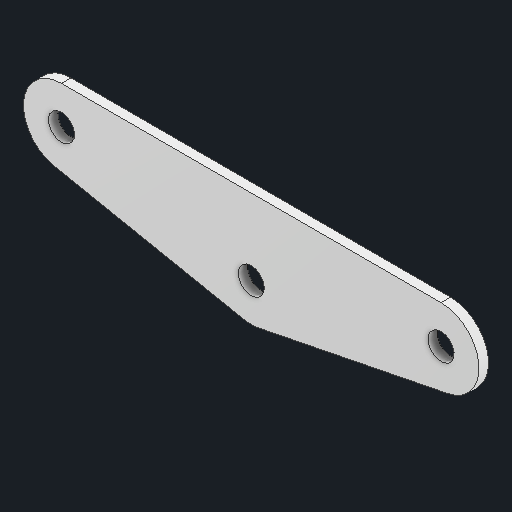
# Autodesk Inventor part: gearbox_gusset
Saved by Autodesk Inventor 2025 (Build 290162000, 162)
## iProperties
Created: 2024-06-27
Part Number: gearbox_gusset
Material: Acetal Resin, White
Document SubType Name: Modeling
Designer: Averey Ku
Density: 1.425 g/cm^3
Appearance: Smooth - White
Author: Averey Ku
Autodesk Inventor part; units mm, degrees
ref_plane "YZ Plane" through (0, 0, 0) normal (1, 0, 0) x (0, 1, 0)
ref_plane "XZ Plane" through (0, 0, 0) normal (0, 1, 0) x (-1, 0, 0)
ref_plane "XY Plane" through (0, 0, 0) normal (0, 0, 1) x (1, 0, 0)
sketch "main" plane through (0, 0, 0) normal (0, 0, 1) x (1, 0, 0)
  circle A0 centre (5.5393, 31.9986) radius 2.1844
  circle A1 centre (5.5393, -31.5014) radius 2.1844
  arc A2 (11.8893, 31.9986) -> (-0.6874, 33.244) centre (5.5393, 31.9986) ccw
  arc A3 (-0.6874, -32.7467) -> (11.8893, -31.5014) centre (5.5393, -31.5014) ccw
  line L0 (11.8893, 31.9986) -> (11.8893, -31.5014)
  circle A4 centre (-0.8107, 0.2486) radius 2.1844
  arc A5 (-7.0374, 1.494) -> (-7.0374, -0.9967) centre (-0.8107, 0.2486) ccw
  line L1 (-0.6874, 33.244) -> (-7.0374, 1.494)
  line L2 (-7.0374, -0.9967) -> (-0.6874, -32.7467)
  point P0 (2.0663, 0.2486)
sketch "Sketch1" plane through (0, 0, 0) normal (0, 0, 1) x (1, 0, 0)
  circle A0 centre (0, 0) radius 2.1844
  circle A1 centre (63.5, -0.0173) radius 2.1844
  arc A2 (0.0017, 6.35) -> (-1.247, -6.2263) centre (0, 0) ccw
  arc A3 (64.7436, -6.2443) -> (63.5017, 6.3327) centre (63.5, -0.0173) ccw
  line L0 (0.0017, 6.35) -> (63.5017, 6.3327)
  circle A4 centre (31.7483, -6.3586) radius 2.1844
  arc A5 (30.5012, -12.585) -> (32.9919, -12.5857) centre (31.7483, -6.3586) ccw
  line L1 (-1.247, -6.2263) -> (30.5012, -12.585)
  line L2 (32.9919, -12.5857) -> (64.7436, -6.2443)
  point P0 (0, 0)
  constraints: 2 other
extrude "Extrusion1" add sketch "Sketch1" along normal blind 1.5875
body "Solid1"
